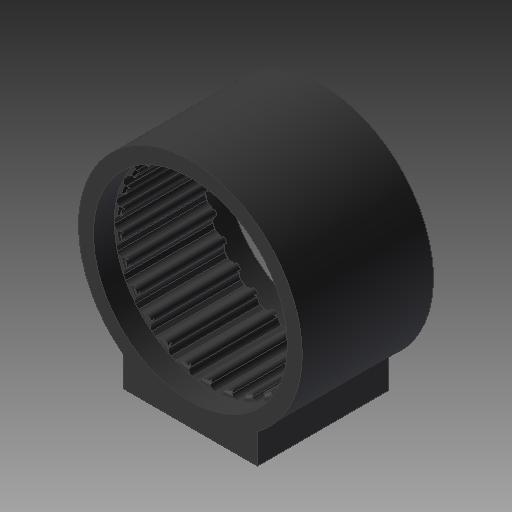
# Autodesk Inventor part: eq_Outer_tri_body_end_6810
Saved by Autodesk Inventor 2017 (Build 210142000, 142)
## iProperties
Created: 2018-11-04
Part Number: eq_Outer_tri_body_end_6810
Material: Generic
Document SubType Name: Modeling
Designer: paulg
Density: 1 g/cm^3
Appearance: Default
Author: paulg
Autodesk Inventor part; units mm, degrees
ref_plane "YZ Plane" through (0, 0, 0) normal (1, 0, 0) x (0, 1, 0)
ref_plane "XZ Plane" through (0, 0, 0) normal (0, 1, 0) x (-1, 0, 0)
ref_plane "XY Plane" through (0, 0, 0) normal (0, 0, 1) x (1, 0, 0)
sketch "Sketch1" plane through (0, 0, 0) normal (0, 0, 1) x (1, 0, 0)
  circle A0 centre (0, 0) radius 37.5
  line L0 (0, 0) -> (31.65, 0)
  circle A1 centre (31.65, 0) radius 1.5
  circle A2 centre (29.8376, 2.9942) radius 2 construction
  circle A3 centre (0, 0) radius 31.15
  line L1 (29.8376, 2.9942) -> (30.9514, 3.5115)
  circle A4 centre (30.7969, 7.299) radius 1.5
  circle A5 centre (28.2835, 14.2045) radius 1.5
  circle A6 centre (24.2453, 20.3442) radius 1.5
  circle A7 centre (18.9001, 25.3872) radius 1.5
  circle A8 centre (12.5359, 29.0615) radius 1.5
  circle A9 centre (5.496, 31.1692) radius 1.5
  circle A10 centre (-1.8403, 31.5965) radius 1.5
  circle A11 centre (-9.0773, 30.3204) radius 1.5
  circle A12 centre (-15.825, 27.4097) radius 1.5
  circle A13 centre (-21.7195, 23.0214) radius 1.5
  circle A14 centre (-26.4432, 17.392) radius 1.5
  circle A15 centre (-29.7413, 10.8249) radius 1.5
  circle A16 centre (-31.436, 3.6743) radius 1.5
  circle A17 centre (-31.436, -3.6743) radius 1.5
  circle A18 centre (-29.7413, -10.8249) radius 1.5
  circle A19 centre (-26.4432, -17.392) radius 1.5
  circle A20 centre (-21.7195, -23.0214) radius 1.5
  circle A21 centre (-15.825, -27.4097) radius 1.5
  circle A22 centre (-9.0773, -30.3204) radius 1.5
  circle A23 centre (-1.8403, -31.5965) radius 1.5
  circle A24 centre (5.496, -31.1692) radius 1.5
  circle A25 centre (12.5359, -29.0615) radius 1.5
  circle A26 centre (18.9001, -25.3872) radius 1.5
  circle A27 centre (24.2453, -20.3442) radius 1.5
  circle A28 centre (28.2835, -14.2045) radius 1.5
  circle A29 centre (30.7969, -7.299) radius 1.5
  dimension "d164" = 62.3
  dimension "d0" = 75
  dimension "d1" = 31.65
  dimension "d2" = 3
  dimension "d165" = 4
  dimension "d172" = 360
  constraints: 29 centre point, 4 end point, 3 coincident, 1 horizontal, 1 tangent, 58 other
  measures "d0" diameter of A0
  measures "d1" distance of L0.start L0.end
  measures "d2" diameter of A1
  measures "d165" diameter of A2
extrude "Extrusion1" add sketch "Sketch1" along normal mid plane 30 contours A0 | A1 A3 L0 | L0 A3 A1 | A3 A1 | A29 A3 | A3 A29 | A4 A3 | A3 A4 | A28 A3 | A3 A28 | A5 A3 | A3 A5 | A27 A3 | A3 A27 | A6 A3 | A3 A6 | A26 A3 | A3 A26 | A7 A3 | A3 A7 | A25 A3 | A3 A25 | A8 A3 | A3 A8 | A24 A3 | A3 A24 | A9 A3 | A3 A9 | A23 A3 | A3 A23 | A10 A3 | A3 A10 | A22 A3 | A3 A22 | A11 A3 | A3 A11 | A21 A3 | A3 A21 | A12 A3 | A3 A12 | A20 A3 | A3 A20 | A13 A3 | A3 A13 | A19 A3 | A3 A19 | A14 A3 | A3 A14 | A18 A3 | A3 A18 | A15 A3 | A3 A15 | A17 A3 | A3 A17 | A16 A3 | A3 A16
sketch "Sketch3" plane through (0, 0, 15) normal (0, 0, 1) x (1, 0, 0)
  circle A0 centre (0, 0) radius 37.5 projected
  arc A1 (31.1184, 1.4026) -> (31.1184, -1.4026) centre (31.65, 0) ccw projected
  arc A2 (30.6031, -5.8116) -> (31.1184, -1.4026) centre (0, 0) ccw projected
  arc A3 (32.3785, 4.5738) -> (32.5606, 3.0165) centre (30.3434, 3.5466) ccw
  line L0 (30.3434, 3.5466) -> (30.9394, 3.6163)
  arc A4 (32.5606, 3.0165) -> (32.3785, 4.5738) centre (0, 0) ccw
  arc A5 (28.4379, -12.7125) -> (27.1789, -15.2194) centre (28.2835, -14.2045) ccw projected
  arc A6 (24.7397, -18.928) -> (27.1789, -15.2194) centre (0, 0) ccw projected
  arc A7 (24.7397, -18.928) -> (22.9365, -21.077) centre (24.2453, -20.3442) ccw projected
  arc A8 (19.7077, -24.1232) -> (22.9365, -21.077) centre (0, 0) ccw projected
  arc A9 (19.7077, -24.1232) -> (17.4575, -25.7984) centre (18.9001, -25.3872) ccw projected
  arc A10 (13.6133, -28.0179) -> (17.4575, -25.7984) centre (0, 0) ccw projected
  arc A11 (13.6133, -28.0179) -> (11.0374, -29.129) centre (12.5359, -29.0615) ccw projected
  arc A12 (6.785, -30.4021) -> (11.0374, -29.129) centre (0, 0) ccw projected
  arc A13 (6.785, -30.4021) -> (4.0223, -30.8892) centre (5.496, -31.1692) ccw projected
  arc A14 (-0.4091, -31.1473) -> (4.0223, -30.8892) centre (0, 0) ccw projected
  arc A15 (-0.4091, -31.1473) -> (-3.2096, -30.9842) centre (-1.8403, -31.5965) ccw projected
  arc A16 (-7.5811, -30.2134) -> (-3.2096, -30.9842) centre (0, 0) ccw projected
  arc A17 (-7.5811, -30.2134) -> (-10.2686, -29.4088) centre (-9.0773, -30.3204) ccw projected
  arc A18 (-14.3445, -27.6507) -> (-10.2686, -29.4088) centre (0, 0) ccw projected
  arc A19 (-14.3445, -27.6507) -> (-16.7739, -26.248) centre (-15.825, -27.4097) ccw projected
  arc A20 (-20.3345, -23.5973) -> (-16.7739, -26.248) centre (0, 0) ccw projected
  arc A21 (-20.3345, -23.5973) -> (-22.375, -21.6722) centre (-21.7195, -23.0214) ccw projected
  arc A22 (-25.2283, -18.2717) -> (-22.375, -21.6722) centre (0, 0) ccw projected
  arc A23 (-25.2283, -18.2717) -> (-26.7698, -15.928) centre (-26.4432, -17.392) ccw projected
  arc A24 (-28.762, -11.9612) -> (-26.7698, -15.928) centre (0, 0) ccw projected
  arc A25 (-28.762, -11.9612) -> (-29.7215, -9.3251) centre (-29.7413, -10.8249) ccw projected
  arc A26 (-30.7452, -5.0058) -> (-29.7215, -9.3251) centre (0, 0) ccw projected
  arc A27 (-30.7452, -5.0058) -> (-31.0708, -2.2195) centre (-31.436, -3.6743) ccw projected
  arc A28 (-31.0708, 2.2195) -> (-31.0708, -2.2195) centre (0, 0) ccw projected
  arc A29 (-31.0708, 2.2195) -> (-30.7452, 5.0058) centre (-31.436, 3.6743) ccw projected
  arc A30 (-29.7215, 9.3251) -> (-30.7452, 5.0058) centre (0, 0) ccw projected
  arc A31 (-29.7215, 9.3251) -> (-28.762, 11.9612) centre (-29.7413, 10.8249) ccw projected
  arc A32 (-26.7698, 15.928) -> (-28.762, 11.9612) centre (0, 0) ccw projected
  arc A33 (-26.7698, 15.928) -> (-25.2283, 18.2717) centre (-26.4432, 17.392) ccw projected
  arc A34 (-22.375, 21.6722) -> (-25.2283, 18.2717) centre (0, 0) ccw projected
  arc A35 (-22.375, 21.6722) -> (-20.3345, 23.5973) centre (-21.7195, 23.0214) ccw projected
  arc A36 (-16.7739, 26.248) -> (-20.3345, 23.5973) centre (0, 0) ccw projected
  arc A37 (-16.7739, 26.248) -> (-14.3445, 27.6507) centre (-15.825, 27.4097) ccw projected
  arc A38 (-10.2686, 29.4088) -> (-14.3445, 27.6507) centre (0, 0) ccw projected
  arc A39 (-10.2686, 29.4088) -> (-7.5811, 30.2134) centre (-9.0773, 30.3204) ccw projected
  arc A40 (-3.2096, 30.9842) -> (-7.5811, 30.2134) centre (0, 0) ccw projected
  arc A41 (-3.2096, 30.9842) -> (-0.4091, 31.1473) centre (-1.8403, 31.5965) ccw projected
  arc A42 (4.0223, 30.8892) -> (-0.4091, 31.1473) centre (0, 0) ccw projected
  arc A43 (4.0223, 30.8892) -> (6.785, 30.4021) centre (5.496, 31.1692) ccw projected
  arc A44 (11.0374, 29.129) -> (6.785, 30.4021) centre (0, 0) ccw projected
  arc A45 (11.0374, 29.129) -> (13.6133, 28.0179) centre (12.5359, 29.0615) ccw projected
  arc A46 (17.4575, 25.7984) -> (13.6133, 28.0179) centre (0, 0) ccw projected
  arc A47 (17.4575, 25.7984) -> (19.7077, 24.1232) centre (18.9001, 25.3872) ccw projected
  arc A48 (22.9365, 21.077) -> (19.7077, 24.1232) centre (0, 0) ccw projected
  arc A49 (22.9365, 21.077) -> (24.7397, 18.928) centre (24.2453, 20.3442) ccw projected
  arc A50 (27.1789, 15.2194) -> (24.7397, 18.928) centre (0, 0) ccw projected
  arc A51 (27.1789, 15.2194) -> (28.4379, 12.7125) centre (28.2835, 14.2045) ccw projected
  arc A52 (29.9561, 8.5412) -> (28.4379, 12.7125) centre (0, 0) ccw projected
  arc A53 (29.9561, 8.5412) -> (30.6031, 5.8116) centre (30.7969, 7.299) ccw projected
  arc A54 (31.1184, 1.4026) -> (30.6031, 5.8116) centre (0, 0) ccw projected
  arc A55 (30.6031, -5.8116) -> (29.9561, -8.5412) centre (30.7969, -7.299) ccw projected
  arc A56 (28.4379, -12.7125) -> (29.9561, -8.5412) centre (0, 0) ccw projected
  dimension "d115" = 0.6
  dimension "d169" = 32.7
  constraints: 5 point on circle, 2 centre point, 2 end point, 2 tangent, 1 coincident
  measures "d115" distance of L0.end L0.start
  measures "d169" radius of A4
extrude "Extrusion3" cut sketch "Sketch3" against normal through all contours A54 A3 A4 | A3 A54
pattern_circular "Circular Pattern1" count 27 over 360 about axis through (0, 0, 0) along (0, 0, 1) of "Extrusion3"
sketch "Sketch16" plane through (0, 0, 15) normal (0, 0, 1) x (1, 0, 0)
  arc A0 (27.7434, -17.3088) -> (27.1789, -15.2195) centre (25.5242, -16.7875) ccw projected
  arc A1 (23.0039, -23.2403) -> (22.9364, -21.0771) centre (20.9647, -22.2213) ccw projected
  arc A2 (17.0243, -27.9189) -> (17.4574, -25.7985) centre (15.275, -26.4571) ccw projected
  arc A3 (10.1268, -31.0924) -> (11.0373, -29.129) centre (8.7618, -29.2666) ccw projected
  arc A4 (2.6835, -32.5897) -> (4.0222, -30.8892) centre (1.7763, -30.4983) ccw projected
  arc A5 (-4.9046, -32.3301) -> (-3.2098, -30.9842) centre (-5.305, -30.0859) ccw projected
  arc A6 (-12.2282, -30.3276) -> (-10.2687, -29.4088) centre (-12.1002, -28.0515) ccw projected
  arc A7 (-18.8926, -26.6901) -> (-16.774, -26.2479) centre (-18.2432, -24.5049) ccw projected
  arc A8 (-24.5385, -21.6137) -> (-22.3751, -21.6721) centre (-23.4027, -19.6372) ccw projected
  arc A9 (-28.8615, -15.3721) -> (-26.7699, -15.9279) centre (-27.3005, -13.7108) ccw projected
  arc A10 (-31.6286, -8.3018) -> (-29.7215, -9.325) centre (-29.7265, -7.0453) ccw projected
  arc A11 (-32.6906, -0.784) -> (-31.0708, -2.2194) centre (-30.55, 0) ccw projected
  arc A12 (-31.9902, 6.7761) -> (-30.7451, 5.0059) centre (-29.7265, 7.0453) ccw projected
  arc A13 (-29.5652, 13.9709) -> (-28.762, 11.9613) centre (-27.3005, 13.7108) ccw projected
  arc A14 (-25.5464, 20.4125) -> (-25.2282, 18.2718) centre (-23.4027, 19.6372) ccw projected
  arc A15 (-20.1503, 25.7537) -> (-20.3344, 23.5973) centre (-18.2432, 24.5049) ccw projected
  arc A16 (-13.668, 29.7065) -> (-14.3444, 27.6507) centre (-12.1002, 28.0515) ccw projected
  arc A17 (-6.4487, 32.0578) -> (-7.581, 30.2134) centre (-5.305, 30.0859) ccw projected
  arc A18 (1.1181, 32.6809) -> (-0.409, 31.1473) centre (1.7763, 30.4983) ccw projected
  arc A19 (8.6247, 31.5421) -> (6.7851, 30.4021) centre (8.7618, 29.2666) ccw projected
  arc A20 (15.6663, 28.7029) -> (13.6134, 28.0178) centre (15.275, 26.4571) ccw projected
  arc A21 (21.8634, 24.3163) -> (19.7078, 24.1231) centre (20.9647, 22.2213) ccw projected
  arc A22 (26.8818, 18.6188) -> (24.7398, 18.9279) centre (25.5242, 16.7875) ccw projected
  arc A23 (30.451, 11.9176) -> (28.438, 12.7124) centre (28.7076, 10.4487) ccw projected
  arc A24 (31.1184, 1.4028) -> (32.5606, 3.0165) centre (30.3434, 3.5466) ccw projected
  arc A25 (31.1184, 1.4026) -> (31.1184, -1.4026) centre (31.65, 0) ccw projected
  circle A26 centre (0, 0) radius 37.5 projected
  line L0 (0, 0) -> (35, 0)
  circle A27 centre (35, 0) radius 1.25
  arc A28 (30.9873, -10.4441) -> (29.9561, -8.5413) centre (28.7076, -10.4487) ccw projected
  arc A29 (30.451, -11.9176) -> (30.9873, -10.4441) centre (0, 0) ccw projected
  arc A30 (26.8818, -18.6188) -> (27.7434, -17.3088) centre (0, 0) ccw projected
  arc A31 (21.8634, -24.3163) -> (23.0039, -23.2403) centre (0, 0) ccw projected
  arc A32 (15.6663, -28.7029) -> (17.0243, -27.9189) centre (0, 0) ccw projected
  arc A33 (8.6247, -31.5421) -> (10.1268, -31.0924) centre (0, 0) ccw projected
  arc A34 (1.1181, -32.6809) -> (2.6835, -32.5897) centre (0, 0) ccw projected
  arc A35 (-6.4487, -32.0578) -> (-4.9046, -32.3301) centre (0, 0) ccw projected
  arc A36 (-13.668, -29.7065) -> (-12.2282, -30.3276) centre (0, 0) ccw projected
  arc A37 (-20.1503, -25.7537) -> (-18.8926, -26.6901) centre (0, 0) ccw projected
  arc A38 (-25.5464, -20.4125) -> (-24.5385, -21.6137) centre (0, 0) ccw projected
  arc A39 (-29.5652, -13.9709) -> (-28.8615, -15.3721) centre (0, 0) ccw projected
  arc A40 (-31.9902, -6.7761) -> (-31.6286, -8.3018) centre (0, 0) ccw projected
  arc A41 (-32.6906, 0.784) -> (-32.6906, -0.784) centre (0, 0) ccw projected
  arc A42 (-31.6286, 8.3018) -> (-31.9902, 6.7761) centre (0, 0) ccw projected
  arc A43 (-28.8615, 15.3721) -> (-29.5652, 13.9709) centre (0, 0) ccw projected
  arc A44 (-24.5385, 21.6137) -> (-25.5464, 20.4125) centre (0, 0) ccw projected
  arc A45 (-18.8926, 26.6901) -> (-20.1503, 25.7537) centre (0, 0) ccw projected
  arc A46 (-12.2282, 30.3276) -> (-13.668, 29.7065) centre (0, 0) ccw projected
  arc A47 (-4.9046, 32.3301) -> (-6.4487, 32.0578) centre (0, 0) ccw projected
  arc A48 (2.6835, 32.5897) -> (1.1181, 32.6809) centre (0, 0) ccw projected
  arc A49 (10.1268, 31.0924) -> (8.6247, 31.5421) centre (0, 0) ccw projected
  arc A50 (17.0243, 27.9189) -> (15.6663, 28.7029) centre (0, 0) ccw projected
  arc A51 (23.0039, 23.2403) -> (21.8634, 24.3163) centre (0, 0) ccw projected
  arc A52 (27.7434, 17.3088) -> (26.8818, 18.6188) centre (0, 0) ccw projected
  arc A53 (30.9873, 10.4441) -> (30.451, 11.9176) centre (0, 0) ccw projected
  arc A54 (32.5606, 3.0165) -> (32.3785, 4.5738) centre (0, 0) ccw projected
  arc A55 (28.4379, -12.7125) -> (27.1789, -15.2194) centre (28.2835, -14.2045) ccw projected
  arc A56 (24.7397, -18.928) -> (22.9365, -21.077) centre (24.2453, -20.3442) ccw projected
  arc A57 (19.7077, -24.1232) -> (17.4575, -25.7984) centre (18.9001, -25.3872) ccw projected
  arc A58 (13.6133, -28.0179) -> (11.0374, -29.129) centre (12.5359, -29.0615) ccw projected
  arc A59 (6.785, -30.4021) -> (4.0223, -30.8892) centre (5.496, -31.1692) ccw projected
  arc A60 (-0.4091, -31.1473) -> (-3.2096, -30.9842) centre (-1.8403, -31.5965) ccw projected
  arc A61 (-7.5811, -30.2134) -> (-10.2686, -29.4088) centre (-9.0773, -30.3204) ccw projected
  arc A62 (-14.3445, -27.6507) -> (-16.7739, -26.248) centre (-15.825, -27.4097) ccw projected
  arc A63 (-20.3345, -23.5973) -> (-22.375, -21.6722) centre (-21.7195, -23.0214) ccw projected
  arc A64 (-25.2283, -18.2717) -> (-26.7698, -15.928) centre (-26.4432, -17.392) ccw projected
  arc A65 (-28.762, -11.9612) -> (-29.7215, -9.3251) centre (-29.7413, -10.8249) ccw projected
  arc A66 (-30.7452, -5.0058) -> (-31.0708, -2.2195) centre (-31.436, -3.6743) ccw projected
  arc A67 (-31.0708, 2.2195) -> (-30.7452, 5.0058) centre (-31.436, 3.6743) ccw projected
  arc A68 (-29.7215, 9.3251) -> (-28.762, 11.9612) centre (-29.7413, 10.8249) ccw projected
  arc A69 (-26.7698, 15.928) -> (-25.2283, 18.2717) centre (-26.4432, 17.392) ccw projected
  arc A70 (-22.375, 21.6722) -> (-20.3345, 23.5973) centre (-21.7195, 23.0214) ccw projected
  arc A71 (-16.7739, 26.248) -> (-14.3445, 27.6507) centre (-15.825, 27.4097) ccw projected
  arc A72 (-10.2686, 29.4088) -> (-7.5811, 30.2134) centre (-9.0773, 30.3204) ccw projected
  arc A73 (-3.2096, 30.9842) -> (-0.4091, 31.1473) centre (-1.8403, 31.5965) ccw projected
  arc A74 (4.0223, 30.8892) -> (6.785, 30.4021) centre (5.496, 31.1692) ccw projected
  arc A75 (11.0374, 29.129) -> (13.6133, 28.0179) centre (12.5359, 29.0615) ccw projected
  arc A76 (17.4575, 25.7984) -> (19.7077, 24.1232) centre (18.9001, 25.3872) ccw projected
  arc A77 (22.9365, 21.077) -> (24.7397, 18.928) centre (24.2453, 20.3442) ccw projected
  arc A78 (27.1789, 15.2194) -> (28.4379, 12.7125) centre (28.2835, 14.2045) ccw projected
  arc A79 (29.9561, 8.5412) -> (30.6031, 5.8116) centre (30.7969, 7.299) ccw projected
  arc A80 (28.4379, -12.7125) -> (28.438, -12.7124) centre (0, 0) ccw projected
  arc A81 (27.1789, -15.2195) -> (27.1789, -15.2194) centre (0, 0) ccw projected
  arc A82 (24.7398, -18.9279) -> (26.8818, -18.6188) centre (25.5242, -16.7875) ccw projected
  arc A83 (24.7397, -18.928) -> (24.7398, -18.9279) centre (0, 0) ccw projected
  arc A84 (22.9364, -21.0771) -> (22.9365, -21.077) centre (0, 0) ccw projected
  arc A85 (19.7078, -24.1231) -> (21.8634, -24.3163) centre (20.9647, -22.2213) ccw projected
  arc A86 (19.7077, -24.1232) -> (19.7078, -24.1231) centre (0, 0) ccw projected
  arc A87 (17.4574, -25.7985) -> (17.4575, -25.7984) centre (0, 0) ccw projected
  arc A88 (13.6134, -28.0178) -> (15.6663, -28.7029) centre (15.275, -26.4571) ccw projected
  arc A89 (13.6133, -28.0179) -> (13.6134, -28.0178) centre (0, 0) ccw projected
  arc A90 (11.0373, -29.129) -> (11.0374, -29.129) centre (0, 0) ccw projected
  arc A91 (6.7851, -30.4021) -> (8.6247, -31.5421) centre (8.7618, -29.2666) ccw projected
  arc A92 (6.785, -30.4021) -> (6.7851, -30.4021) centre (0, 0) ccw projected
  arc A93 (4.0222, -30.8892) -> (4.0223, -30.8892) centre (0, 0) ccw projected
  arc A94 (-0.409, -31.1473) -> (1.1181, -32.6809) centre (1.7763, -30.4983) ccw projected
  arc A95 (-0.4091, -31.1473) -> (-0.409, -31.1473) centre (0, 0) ccw projected
  arc A96 (-3.2098, -30.9842) -> (-3.2096, -30.9842) centre (0, 0) ccw projected
  arc A97 (-7.581, -30.2134) -> (-6.4487, -32.0578) centre (-5.305, -30.0859) ccw projected
  arc A98 (-7.5811, -30.2134) -> (-7.581, -30.2134) centre (0, 0) ccw projected
  arc A99 (-10.2687, -29.4088) -> (-10.2686, -29.4088) centre (0, 0) ccw projected
  arc A100 (-14.3444, -27.6507) -> (-13.668, -29.7065) centre (-12.1002, -28.0515) ccw projected
  arc A101 (-14.3445, -27.6507) -> (-14.3444, -27.6507) centre (0, 0) ccw projected
  arc A102 (-16.774, -26.2479) -> (-16.7739, -26.248) centre (0, 0) ccw projected
  arc A103 (-20.3344, -23.5973) -> (-20.1503, -25.7537) centre (-18.2432, -24.5049) ccw projected
  arc A104 (-20.3345, -23.5973) -> (-20.3344, -23.5973) centre (0, 0) ccw projected
  arc A105 (-22.3751, -21.6721) -> (-22.375, -21.6722) centre (0, 0) ccw projected
  arc A106 (-25.2282, -18.2718) -> (-25.5464, -20.4125) centre (-23.4027, -19.6372) ccw projected
  arc A107 (-25.2283, -18.2717) -> (-25.2282, -18.2718) centre (0, 0) ccw projected
  arc A108 (-26.7699, -15.9279) -> (-26.7698, -15.928) centre (0, 0) ccw projected
  arc A109 (-28.762, -11.9613) -> (-29.5652, -13.9709) centre (-27.3005, -13.7108) ccw projected
  arc A110 (-28.762, -11.9612) -> (-28.762, -11.9613) centre (0, 0) ccw projected
  arc A111 (-29.7215, -9.325) -> (-29.7215, -9.3251) centre (0, 0) ccw projected
  arc A112 (-30.7451, -5.0059) -> (-31.9902, -6.7761) centre (-29.7265, -7.0453) ccw projected
  arc A113 (-30.7452, -5.0058) -> (-30.7451, -5.0059) centre (0, 0) ccw projected
  arc A114 (-31.0708, -2.2194) -> (-31.0708, -2.2195) centre (0, 0) ccw projected
  arc A115 (-31.0708, 2.2194) -> (-32.6906, 0.784) centre (-30.55, 0) ccw projected
  arc A116 (-31.0708, 2.2195) -> (-31.0708, 2.2194) centre (0, 0) ccw projected
  arc A117 (-30.7451, 5.0059) -> (-30.7452, 5.0058) centre (0, 0) ccw projected
  arc A118 (-29.7215, 9.325) -> (-31.6286, 8.3018) centre (-29.7265, 7.0453) ccw projected
  arc A119 (-29.7215, 9.3251) -> (-29.7215, 9.325) centre (0, 0) ccw projected
  arc A120 (-28.762, 11.9613) -> (-28.762, 11.9612) centre (0, 0) ccw projected
  arc A121 (-26.7699, 15.9279) -> (-28.8615, 15.3721) centre (-27.3005, 13.7108) ccw projected
  arc A122 (-26.7698, 15.928) -> (-26.7699, 15.9279) centre (0, 0) ccw projected
  arc A123 (-25.2282, 18.2718) -> (-25.2283, 18.2717) centre (0, 0) ccw projected
  arc A124 (-22.3751, 21.6721) -> (-24.5385, 21.6137) centre (-23.4027, 19.6372) ccw projected
  arc A125 (-22.375, 21.6722) -> (-22.3751, 21.6721) centre (0, 0) ccw projected
  arc A126 (-20.3344, 23.5973) -> (-20.3345, 23.5973) centre (0, 0) ccw projected
  arc A127 (-16.774, 26.2479) -> (-18.8926, 26.6901) centre (-18.2432, 24.5049) ccw projected
  arc A128 (-16.7739, 26.248) -> (-16.774, 26.2479) centre (0, 0) ccw projected
  arc A129 (-14.3444, 27.6507) -> (-14.3445, 27.6507) centre (0, 0) ccw projected
  arc A130 (-10.2687, 29.4088) -> (-12.2282, 30.3276) centre (-12.1002, 28.0515) ccw projected
  arc A131 (-10.2686, 29.4088) -> (-10.2687, 29.4088) centre (0, 0) ccw projected
  arc A132 (-7.581, 30.2134) -> (-7.5811, 30.2134) centre (0, 0) ccw projected
  arc A133 (-3.2098, 30.9842) -> (-4.9046, 32.3301) centre (-5.305, 30.0859) ccw projected
  arc A134 (-3.2096, 30.9842) -> (-3.2098, 30.9842) centre (0, 0) ccw projected
  arc A135 (-0.409, 31.1473) -> (-0.4091, 31.1473) centre (0, 0) ccw projected
  arc A136 (4.0222, 30.8892) -> (2.6835, 32.5897) centre (1.7763, 30.4983) ccw projected
  arc A137 (4.0223, 30.8892) -> (4.0222, 30.8892) centre (0, 0) ccw projected
  arc A138 (6.7851, 30.4021) -> (6.785, 30.4021) centre (0, 0) ccw projected
  arc A139 (11.0373, 29.129) -> (10.1268, 31.0924) centre (8.7618, 29.2666) ccw projected
  arc A140 (11.0374, 29.129) -> (11.0373, 29.129) centre (0, 0) ccw projected
  arc A141 (13.6134, 28.0178) -> (13.6133, 28.0179) centre (0, 0) ccw projected
  arc A142 (17.4574, 25.7985) -> (17.0243, 27.9189) centre (15.275, 26.4571) ccw projected
  arc A143 (17.4575, 25.7984) -> (17.4574, 25.7985) centre (0, 0) ccw projected
  arc A144 (19.7078, 24.1231) -> (19.7077, 24.1232) centre (0, 0) ccw projected
  arc A145 (22.9364, 21.0771) -> (23.0039, 23.2403) centre (20.9647, 22.2213) ccw projected
  arc A146 (22.9365, 21.077) -> (22.9364, 21.0771) centre (0, 0) ccw projected
  arc A147 (24.7398, 18.9279) -> (24.7397, 18.928) centre (0, 0) ccw projected
  arc A148 (27.1789, 15.2195) -> (27.7434, 17.3088) centre (25.5242, 16.7875) ccw projected
  arc A149 (27.1789, 15.2194) -> (27.1789, 15.2195) centre (0, 0) ccw projected
  arc A150 (28.438, 12.7124) -> (28.4379, 12.7125) centre (0, 0) ccw projected
  arc A151 (29.9561, 8.5413) -> (30.9873, 10.4441) centre (28.7076, 10.4487) ccw projected
  arc A152 (29.9561, 8.5412) -> (29.9561, 8.5413) centre (0, 0) ccw projected
  arc A153 (30.6031, 5.8115) -> (30.6031, 5.8116) centre (0, 0) ccw projected
  arc A154 (32.3785, 4.5738) -> (30.6031, 5.8115) centre (30.3434, 3.5466) ccw projected
  arc A155 (31.1184, 1.4026) -> (31.1184, 1.4028) centre (0, 0) ccw projected
  arc A156 (30.6031, -5.8116) -> (30.6031, -5.8115) centre (0, 0) ccw projected
  arc A157 (32.5606, -3.0165) -> (31.1184, -1.4028) centre (30.3434, -3.5466) ccw projected
  arc A158 (32.3785, -4.5738) -> (32.5606, -3.0165) centre (0, 0) ccw projected
  arc A159 (30.6031, -5.8115) -> (32.3785, -4.5738) centre (30.3434, -3.5466) ccw projected
  arc A160 (28.438, -12.7124) -> (30.451, -11.9176) centre (28.7076, -10.4487) ccw projected
  arc A161 (30.6031, -5.8116) -> (29.9561, -8.5412) centre (30.7969, -7.299) ccw projected
  arc A162 (29.9561, -8.5413) -> (29.9561, -8.5412) centre (0, 0) ccw projected
  arc A163 (31.1184, -1.4028) -> (31.1184, -1.4026) centre (0, 0) ccw projected
  point P0 (13.8628, 32.1376)
  point P1 (-24.0185, 25.4581)
  point P2 (-32.8892, -11.9707)
  point P3 (-2.0351, -34.9408)
  point P4 (31.2771, -15.708)
  dimension "d100" = 2.5
  dimension "d101" = 35
  dimension "d104" = 333.333
  constraints: 2 coincident, 2 end point, 1 centre point, 1 horizontal, 6 other
  measures "d100" diameter of A27
  measures "d101" distance of L0.start L0.end
hole "Hole4" [suppressed]
sketch "Sketch17" plane through (0, 0, -15) normal (0, 0, -1) x (-1, 0, 0)
  circle A0 centre (0, 0) radius 37.5 projected
  circle A1 centre (0, 0) radius 32.5
  dimension "d116" = 65
  constraints: 1 centre point, 1 coincident
  measures "d116" diameter of A1
extrude "Extrusion11" add sketch "Sketch17" along normal blind 7
sketch "Sketch24" plane through (0, 0, 15) normal (0, 0, 1) x (1, 0, 0)
  circle A0 centre (0, 0) radius 32.5
  circle A1 centre (0, 0) radius 37.5 projected
  dimension "d166" = 65
  constraints: 1 centre point, 1 coincident
  measures "d166" diameter of A0
extrude "Extrusion17" add sketch "Sketch24" along normal blind 7
sketch "Sketch25" plane through (0, 0, 0) normal (0, 0, 1) x (1, 0, 0)
  circle A0 centre (0, 0) radius 37.5 projected
  circle A1 centre (0, 0) radius 37.5 projected
  line L0 (0, 0) -> (0, -35) construction
  line L1 (22.5, -40) -> (-22.5, -40)
  line L2 (-22.5, -40) -> (-22.5, -30)
  line L3 (-22.5, -30) -> (22.5, -30) construction
  line L4 (22.5, -30) -> (22.5, -40)
  line L5 (22.5, -40) -> (-22.5, -30) construction
  line L6 (-22.5, -40) -> (22.5, -30) construction
  arc A2 (-22.5, -30) -> (22.5, -30) centre (0, 0) ccw
  dimension "d174" = 45
  dimension "d175" = 40
  constraints: 14 end point, 2 midpoint, 2 parallel, 2 point on circle, 1 centre point, 1 coincident, 1 horizontal, 1 perpendicular, 1 vertical, 4 other
  measures "d174" distance of L1.start L1.end
  measures "d175" distance from line of L1 point (0, 0)
extrude "Extrusion18" add sketch "Sketch25" against normal up to surface (44 mm away) from surface at 22 contours A0 L4 L1 L2
fillet "Fillet5" [suppressed]
sketch "Sketch27" plane through (0, 0, 0) normal (1, 0, 0) x (0, 1, 0)
  line L0 (-32.5, 22) -> (32.5, 22) projected
  line L1 (-2.5609, 15) -> (2.5609, 15) projected
  line L2 (-4.9798, 15) -> (-2.5609, 15) projected
  line L3 (-9.9636, 15) -> (-4.9798, 15) projected
  line L4 (-12.2521, 15) -> (-9.9636, 15) projected
  line L5 (-16.8291, 15) -> (-12.2521, 15) projected
  line L6 (-18.8639, 15) -> (-16.8291, 15) projected
  line L7 (-22.7874, 15) -> (-18.8639, 15) projected
  line L8 (-24.4587, 15) -> (-22.7874, 15) projected
  line L9 (-27.5172, 15) -> (-24.4587, 15) projected
  line L10 (-28.7349, 15) -> (-27.5172, 15) projected
  line L11 (-30.7636, 15) -> (-28.7349, 15) projected
  line L12 (-31.462, 15) -> (-30.7636, 15) projected
  line L13 (-32.3514, 15) -> (-31.462, 15) projected
  line L14 (-32.493, 15) -> (-32.3514, 15) projected
  line L15 (-32.1952, 15) -> (-32.493, 15) projected
  line L16 (-31.7723, 15) -> (-32.1952, 15) projected
  line L17 (-30.3034, 15) -> (-31.7723, 15) projected
  line L18 (-29.3388, 15) -> (-30.3034, 15) projected
  line L19 (-26.7779, 15) -> (-29.3388, 15) projected
  line L20 (-25.3235, 15) -> (-26.7779, 15) projected
  line L21 (-21.8087, 15) -> (-25.3235, 15) projected
  line L22 (-19.9431, 15) -> (-21.8087, 15) projected
  line L23 (-15.6639, 15) -> (-19.9431, 15) projected
  line L24 (-13.4876, 15) -> (-15.6639, 15) projected
  line L25 (-8.6746, 15) -> (-13.4876, 15) projected
  line L26 (-6.3049, 15) -> (-8.6746, 15) projected
  line L27 (-1.2177, 15) -> (-6.3049, 15) projected
  line L28 (1.2177, 15) -> (-1.2177, 15) projected
  line L29 (6.3049, 15) -> (1.2177, 15) projected
  line L30 (8.6746, 15) -> (6.3049, 15) projected
  line L31 (13.4876, 15) -> (8.6746, 15) projected
  line L32 (15.6639, 15) -> (13.4876, 15) projected
  line L33 (19.9431, 15) -> (15.6639, 15) projected
  line L34 (21.8087, 15) -> (19.9431, 15) projected
  line L35 (25.3235, 15) -> (21.8087, 15) projected
  line L36 (26.7779, 15) -> (25.3235, 15) projected
  line L37 (29.3388, 15) -> (26.7779, 15) projected
  line L38 (30.3034, 15) -> (29.3388, 15) projected
  line L39 (31.7723, 15) -> (30.3034, 15) projected
  line L40 (32.1952, 15) -> (31.7723, 15) projected
  line L41 (32.493, 15) -> (32.1952, 15) projected
  line L42 (32.3514, 15) -> (32.493, 15) projected
  line L43 (31.462, 15) -> (32.3514, 15) projected
  line L44 (30.7636, 15) -> (31.462, 15) projected
  line L45 (28.7349, 15) -> (30.7636, 15) projected
  line L46 (27.5172, 15) -> (28.7349, 15) projected
  line L47 (24.4587, 15) -> (27.5172, 15) projected
  line L48 (22.7874, 15) -> (24.4587, 15) projected
  line L49 (18.8639, 15) -> (22.7874, 15) projected
  line L50 (16.8291, 15) -> (18.8639, 15) projected
  line L51 (12.2521, 15) -> (16.8291, 15) projected
  line L52 (9.9636, 15) -> (12.2521, 15) projected
  line L53 (4.9798, 15) -> (9.9636, 15) projected
  line L54 (2.5609, 15) -> (4.9798, 15) projected
  line L55 (32.5, -22) -> (-32.5, -22) projected
  line L56 (-1.2177, -15) -> (1.2177, -15) projected
  line L57 (-6.3049, -15) -> (-1.2177, -15) projected
  line L58 (-8.6746, -15) -> (-6.3049, -15) projected
  line L59 (-13.4876, -15) -> (-8.6746, -15) projected
  line L60 (-15.6639, -15) -> (-13.4876, -15) projected
  line L61 (-19.9431, -15) -> (-15.6639, -15) projected
  line L62 (-21.8087, -15) -> (-19.9431, -15) projected
  line L63 (-25.3235, -15) -> (-21.8087, -15) projected
  line L64 (-26.7779, -15) -> (-25.3235, -15) projected
  line L65 (-29.3388, -15) -> (-26.7779, -15) projected
  line L66 (-30.3034, -15) -> (-29.3388, -15) projected
  line L67 (-31.7723, -15) -> (-30.3034, -15) projected
  line L68 (-32.1952, -15) -> (-31.7723, -15) projected
  line L69 (-32.493, -15) -> (-32.1952, -15) projected
  line L70 (-32.3514, -15) -> (-32.493, -15) projected
  line L71 (-31.462, -15) -> (-32.3514, -15) projected
  line L72 (-30.7636, -15) -> (-31.462, -15) projected
  line L73 (-28.7349, -15) -> (-30.7636, -15) projected
  line L74 (-27.5172, -15) -> (-28.7349, -15) projected
  line L75 (-24.4587, -15) -> (-27.5172, -15) projected
  line L76 (-22.7874, -15) -> (-24.4587, -15) projected
  line L77 (-18.8639, -15) -> (-22.7874, -15) projected
  line L78 (-16.8291, -15) -> (-18.8639, -15) projected
  line L79 (-12.2521, -15) -> (-16.8291, -15) projected
  line L80 (-9.9636, -15) -> (-12.2521, -15) projected
  line L81 (-4.9798, -15) -> (-9.9636, -15) projected
  line L82 (-2.5609, -15) -> (-4.9798, -15) projected
  line L83 (2.5609, -15) -> (-2.5609, -15) projected
  line L84 (4.9798, -15) -> (2.5609, -15) projected
  line L85 (9.9636, -15) -> (4.9798, -15) projected
  line L86 (12.2521, -15) -> (9.9636, -15) projected
  line L87 (16.8291, -15) -> (12.2521, -15) projected
  line L88 (18.8639, -15) -> (16.8291, -15) projected
  line L89 (22.7874, -15) -> (18.8639, -15) projected
  line L90 (24.4587, -15) -> (22.7874, -15) projected
  line L91 (27.5172, -15) -> (24.4587, -15) projected
  line L92 (28.7349, -15) -> (27.5172, -15) projected
  line L93 (30.7636, -15) -> (28.7349, -15) projected
  line L94 (31.462, -15) -> (30.7636, -15) projected
  line L95 (32.3514, -15) -> (31.462, -15) projected
  line L96 (32.493, -15) -> (32.3514, -15) projected
  line L97 (32.1952, -15) -> (32.493, -15) projected
  line L98 (31.7723, -15) -> (32.1952, -15) projected
  line L99 (30.3034, -15) -> (31.7723, -15) projected
  line L100 (29.3388, -15) -> (30.3034, -15) projected
  line L101 (26.7779, -15) -> (29.3388, -15) projected
  line L102 (25.3235, -15) -> (26.7779, -15) projected
  line L103 (21.8087, -15) -> (25.3235, -15) projected
  line L104 (19.9431, -15) -> (21.8087, -15) projected
  line L105 (15.6639, -15) -> (19.9431, -15) projected
  line L106 (13.4876, -15) -> (15.6639, -15) projected
  line L107 (8.6746, -15) -> (13.4876, -15) projected
  line L108 (6.3049, -15) -> (8.6746, -15) projected
  line L109 (1.2177, -15) -> (6.3049, -15) projected
  line L110 (32.493, 15) -> (32.1952, 15) projected
  line L111 (32.493, 15) -> (30.493, 15)
  line L112 (30.493, 15) -> (30.493, 14)
  line L113 (30.493, 14) -> (31.493, 15)
  line L114 (0, 0) -> (0, 29.5496)
  dimension "d186" = 2
  dimension "d187" = 1
  dimension "d188" = 45
  constraints: 8 end point, 2 vertical, 1 midpoint, 1 point on line
  measures "d186" distance from line of L41.start L112
  measures "d187" distance of L111.end L112.end
  measures "d188" angle of L113 L112
revolve "Revolution1" cut sketch "Sketch27" angle 360 about axis through (0, 0, 0) along (0, 0, 1)
mirror "Mirror1" about plane through (0, 0, 0) normal (0, 0, 1) of "Revolution1"
sketch "Sketch28" plane through (-22.5, -40, -22) normal (0, -1, 0) x (1, 0, 0)
  line L0 (45, 0) -> (0, 0) projected
  line L1 (45, 0) -> (45, 44) projected
  line L2 (45, 44) -> (0, 44) projected
  line L3 (0, 44) -> (0, 0) projected
  line L4 (5, 4.5) -> (40, 4.5) construction
  line L5 (40, 4.5) -> (40, 39.5) construction
  line L6 (40, 39.5) -> (5, 39.5) construction
  line L7 (5, 39.5) -> (5, 4.5) construction
  line L8 (5, 4.5) -> (40, 39.5) construction
  line L9 (40, 4.5) -> (5, 39.5) construction
  point P0 (22.5, 22)
  dimension "d190" = 35
  dimension "d191" = 35
  constraints: 12 end point, 4 coincident, 2 midpoint, 2 parallel, 1 horizontal, 1 perpendicular
  measures "d190" distance of L5.end L6.end
  measures "d191" distance of L4.end L5.end
hole "Hole6" at (17.5, -40, 17.5) at (17.5, -40, -17.5) at (-17.5, -40, 17.5) at (-17.5, -40, -17.5) direction (0, 1, 0) diameter 2.5 depth 8 tip angle 118
equation "\"d2\" = 2 * Rr_"
equation "\"R_\" = 31.5"
equation "\"Rr_\" = 1.5"
equation "\"E_\" = 1"
body "Solid1"
